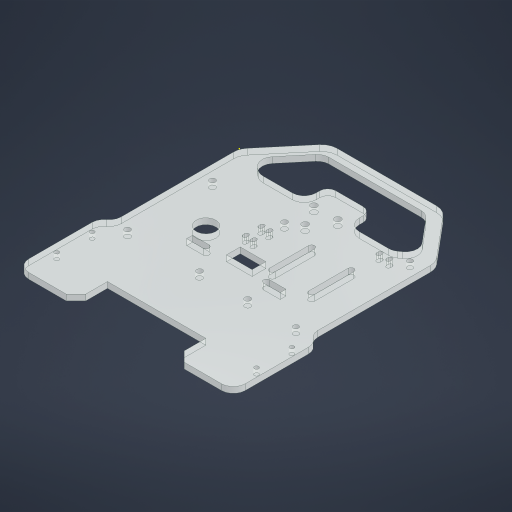
# Autodesk Inventor part: ROBOT CHASSIS PLATE
Saved by Autodesk Inventor 2023 (Build 270158000, 158)
## iProperties
Created: 2023-03-03
Part Number: ROBOT CHASSIS PLATE
Material: Generic
Document SubType Name: Modeling
Designer: Phoenix
Density: 1 g/cm^3
Appearance: Clear
Author: Phoenix
Autodesk Inventor part; units mm, degrees
note: some values were not read from the file. Chosen so that the rebuilt part matches the saved one: sketch regions of "Extrusion1"; arc direction of "Extrusion1".
ref_plane "YZ Plane" through (0, 0, 0) normal (1, 0, 0) x (0, 1, 0)
ref_plane "XZ Plane" through (0, 0, 0) normal (0, 1, 0) x (-1, 0, 0)
ref_plane "XY Plane" through (0, 0, 0) normal (0, 0, 1) x (1, 0, 0)
sketch "Sketch1" plane through (0, 0, 0) normal (0, 1, 0) x (-1, 0, 0)
  line L0 (0, 0) -> (-100, 0) construction
  line L1 (-100, 0) -> (-100, 100)
  line L2 (-100, 100) -> (0, 100)
  line L3 (0, 100) -> (0, 0)
  circle A0 centre (0.75, 92) radius 1.1
  circle A1 centre (0.75, 74) radius 1.1
  line L4 (-50, 100) -> (-50, 0) construction
  line L5 (-7.212, 20.82) -> (-7.212, 64) construction
  line L6 (-7.212, 64) -> (-43.788, 64) construction
  line L7 (-7.212, 20.82) -> (-43.788, 20.82) construction
  circle A2 centre (-7.212, 64) radius 1.5
  circle A3 centre (-43.788, 64) radius 1.5
  circle A4 centre (-7.212, 20.82) radius 1.5
  circle A5 centre (-43.788, 20.82) radius 1.5
  line L8 (-43.788, 6) -> (-92.788, 6) construction
  line L9 (-92.788, 6) -> (-92.788, 64) construction
  line L10 (-92.788, 64) -> (-43.788, 64) construction
  line L11 (-43.788, 64) -> (-43.788, 6) construction
  circle A6 centre (-43.788, 6) radius 1.375
  circle A7 centre (-92.788, 6) radius 1.375
  circle A8 centre (-92.788, 64) radius 1.375
  circle A9 centre (-43.788, 64) radius 1.375
  line L12 (-7.212, 42.41) -> (0, 42.41) construction
  line L13 (-92.788, 35) -> (-100, 35) construction
  line L14 (0, 0) -> (-100, 0) construction
  circle A10 centre (-100.75, 74) radius 1.1
  circle A11 centre (-100.75, 92) radius 1.1
  line L15 (-39, 6) -> (-61, 6)
  line L16 (-61, 6) -> (-61, -6)
  line L17 (-61, -6) -> (-39, -6)
  line L18 (-39, -6) -> (-39, 6)
  line L19 (-39, 6) -> (-61, -6) construction
  line L20 (-61, 6) -> (-39, -6) construction
  line L21 (-50, 0) -> (-50, -25) construction
  line L22 (-50, -25) -> (-20.9775, -25)
  line L23 (-20.9775, -25) -> (0, 0)
  line L24 (-7.8324, 0) -> (-23.7753, -19)
  line L25 (-23.7753, -19) -> (-50, -19)
  line L26 (-39, 6) -> (-16.1201, 6)
  line L27 (-16.1201, 6) -> (-7.8324, 0)
  line L28 (-50, -25) -> (-79.0225, -25)
  line L29 (-79.0225, -25) -> (-100, 0)
  line L30 (-92.1676, 0) -> (-76.2247, -19)
  line L31 (-76.2247, -19) -> (-50, -19)
  line L32 (-61, 6) -> (-83.8799, 6)
  line L33 (-83.8799, 6) -> (-92.1676, 0)
  line L34 (-30, 100) -> (-70, 100)
  line L35 (-50, -1) -> (-50, 12.462) construction
  circle A12 centre (-50, -1) radius 1.15 construction
  circle A13 centre (-50, 12.462) radius 1.15 construction
  circle A14 centre (-50, 9.5) radius 7 construction
  circle A15 centre (-50, 16.5) radius 1.65
  line L36 (0, 100) -> (5, 100)
  line L37 (5, 100) -> (5, 66)
  line L38 (5, 66) -> (0, 66)
  line L39 (0, 66) -> (0, 100)
  line L40 (-100, 100) -> (-105, 100)
  line L41 (-105, 100) -> (-105, 66)
  line L42 (-105, 66) -> (-100, 66)
  line L43 (5, 100) -> (-25, 100)
  line L44 (-25, 100) -> (-25, 108)
  line L45 (-25, 108) -> (5, 108)
  line L46 (5, 108) -> (5, 100)
  line L47 (-75, 100) -> (-75, 108)
  line L48 (-75, 108) -> (-105, 108)
  line L49 (-105, 108) -> (-105, 100)
  line L50 (-25, 100) -> (-75, 100)
  line L51 (-75, 100) -> (-75, 92)
  line L52 (-75, 92) -> (-25, 92)
  line L53 (-25, 92) -> (-25, 100)
  circle A16 centre (-56.0622, 6) radius 1.65
  circle A17 centre (-43.9378, 6) radius 1.65
  point P0 (-50, 80)
  point P1 (-50, 5.731)
  point P2 (-86.6667, 100)
  point P3 (-100, 92.8047)
  point P4 (-100, 91.1953)
  point P5 (-100, 74.8047)
  point P6 (-100, 73.1953)
  point P7 (0, 73.1953)
  point P8 (0, 74.8047)
  point P9 (0, 91.1953)
  point P10 (0, 92.8047)
  dimension "d27" = 3
  dimension "d47" = 14
  dimension "d0" = 100
  dimension "d1" = 100
  dimension "d2" = 8
  dimension "d4" = 2.2
  dimension "d5" = 18
  dimension "d6" = 43.18
  dimension "d7" = 36.576
  dimension "d8" = 3
  dimension "d9" = 49
  dimension "d10" = 58
  dimension "d15" = 2.75
  dimension "d33" = 22
  dimension "d34" = 25
  dimension "d36" = 130
  dimension "d37" = 6
  dimension "d38" = 6
  dimension "d39" = 12
  dimension "d44" = 2.3
  dimension "d45" = 13.462
  dimension "d46" = 5
  dimension "d48" = 15.5
  dimension "d49" = 3.3
  dimension "d55" = 5
  dimension "d56" = 34
  dimension "d57" = 4.25
  dimension "d59" = 30
  dimension "d60" = 8
  dimension "d61" = 8
  dimension "d64" = 360
  constraints: 108 end point, 17 centre point, 15 parallel, 13 symmetric about line, 11 coincident, 11 horizontal, 10 perpendicular, 10 point on line, 8 equal radius, 7 midpoint, 3 vertical, 1 vertical alignment, 11 other
  measures "d0" distance of L1.end L2.end
  measures "d1" distance of L0.end L1.end
  measures "d2" distance from line of L2 point (0.75, 92)
  measures "d4" diameter of A0
  measures "d5" distance of A0.centre A1.centre
  measures "d6" distance of L5.end L5.start
  measures "d7" distance of L5.end L6.end
  measures "d8" diameter of A2
  measures "d9" distance of L6.end L9.end
  measures "d10" distance of L8.end L9.end
  measures "d15" diameter of A8
  measures "d33" distance of L17.end L16.end
  measures "d34" distance of L4.end L21.end
  measures "d36" angle of L0 L23
  measures "d37" distance between parallel lines of L23 L24
  measures "d38" distance between parallel lines of L22 L25
  measures "d39" distance of L17.end L15.start
  measures "d44" diameter of A12
  measures "d45" distance of L35.end L35.start
  measures "d46" distance from line of L17 A12.centre
  measures "d48" distance from line of L17 point (-50, 9.5)
  measures "d49" diameter of A15
  measures "d55" distance of L37.end L38.end
  measures "d56" distance of L36.end L37.end
  measures "d57" distance from line of L37 A0.centre
  measures "d59" distance of L44.end L45.end
  measures "d60" distance of L43.end L44.end
  measures "d61" distance of L51.end L47.start
extrude "Extrusion1" add sketch "Sketch1" along normal blind 3 contours L1 A10 A11 L2 L51 L52 L53 L3 A0 A1 L23 L22 L28 L29 | L42 L41 L40 L1 A11 A10 | L49 L48 L47 L2 L40 | L3 A1 A0 L36 L37 L38 | L36 L2 L44 L45 L46 | L15 L18 L17 L16 A16 A17
fillet "Fillet1" radius 6 8 edges at (61, 1.5, 6) (39, 1.5, 6) (7.8324, 1.5, 0) (92.1676, 1.5, 0) (83.8799, 1.5, 6) (16.1201, 1.5, 6) (23.7753, 1.5, -19) (76.2247, 1.5, -19)
fillet "Fillet1" radius 8 4 edges at (20.9775, 1.5, -25) (0, 1.5, 0) (79.0225, 1.5, -25) (100, 1.5, 0)
fillet "Fillet1" radius 4 2 edges at (61, 1.5, -6) (39, 1.5, -6)
fillet "Fillet1" radius 6 6 edges at (105, 1.5, 66) (100, 1.5, 66) (-5, 1.5, 66) (0, 1.5, 66) (-5, 1.5, 108) (105, 1.5, 108)
sketch "Sketch2" plane through (0, 3, 0) normal (0, 1, 0) x (1, 0, 0)
  point P0 (0, 0)
sketch "Sketch3" plane through (0, 3, 0) normal (0, 1, 0) x (1, 0, 0)
  circle A0 centre (43.788, -64) radius 1.5 projected
  circle A1 centre (92.788, -6) radius 1.375 projected
  line L0 (43.788, -64) -> (92.788, -64) construction
  line L1 (92.788, -64) -> (92.788, -6) construction
  line L2 (92.788, -6) -> (43.788, -6) construction
  line L3 (43.788, -6) -> (43.788, -64) construction
  line L4 (61.788, -25) -> (61.788, -45) construction
  line L5 (60.288, -25) -> (60.288, -45)
  line L6 (63.288, -45) -> (63.288, -25)
  arc A2 (63.288, -25) -> (60.288, -25) centre (61.788, -25) ccw
  arc A3 (60.288, -45) -> (63.288, -45) centre (61.788, -45) ccw
  line L7 (43.788, -35) -> (92.788, -35) construction
  line L8 (81.788, -25) -> (81.788, -45) construction
  line L9 (80.288, -25) -> (80.288, -45)
  line L10 (83.288, -45) -> (83.288, -25)
  arc A4 (83.288, -25) -> (80.288, -25) centre (81.788, -25) ccw
  arc A5 (80.288, -45) -> (83.288, -45) centre (81.788, -45) ccw
  line L11 (63.788, -35) -> (112.788, -35) construction
  line L12 (81.788, -10) -> (81.788, -11) construction
  line L13 (80.788, -10) -> (80.788, -11)
  line L14 (82.788, -11) -> (82.788, -10)
  arc A6 (82.788, -10) -> (80.788, -10) centre (81.788, -10) ccw
  arc A7 (80.788, -11) -> (82.788, -11) centre (81.788, -11) ccw
  line L15 (85.788, -10) -> (85.788, -11)
  arc A8 (85.788, -11) -> (87.788, -11) centre (86.788, -11) ccw
  line L16 (86.788, -10) -> (86.788, -11) construction
  line L17 (87.788, -11) -> (87.788, -10)
  arc A9 (87.788, -10) -> (85.788, -10) centre (86.788, -10) ccw
  line L18 (43.788, -36) -> (43.788, -37) construction
  line L19 (42.788, -36) -> (42.788, -37)
  line L20 (44.788, -37) -> (44.788, -36)
  arc A10 (44.788, -36) -> (42.788, -36) centre (43.788, -36) ccw
  arc A11 (42.788, -37) -> (44.788, -37) centre (43.788, -37) ccw
  line L21 (57, 6) -> (43, 6) construction
  line L22 (50, 6) -> (50, -92) construction
  line L23 (25, -92) -> (75, -92) construction
  line L24 (39.788, -6) -> (39.788, -64) construction
  line L25 (40.788, -37) -> (40.788, -36)
  line L26 (39.788, -36) -> (39.788, -37) construction
  arc A12 (40.788, -36) -> (38.788, -36) centre (39.788, -36) ccw
  line L27 (38.788, -36) -> (38.788, -37)
  arc A13 (38.788, -37) -> (40.788, -37) centre (39.788, -37) ccw
  arc A14 (44.788, -28) -> (42.788, -28) centre (43.788, -28) ccw
  arc A15 (40.788, -28) -> (38.788, -28) centre (39.788, -28) ccw
  line L28 (44.788, -29) -> (44.788, -28)
  arc A16 (42.788, -29) -> (44.788, -29) centre (43.788, -29) ccw
  line L29 (43.788, -28) -> (43.788, -29) construction
  line L30 (42.788, -28) -> (42.788, -29)
  arc A17 (38.788, -29) -> (40.788, -29) centre (39.788, -29) ccw
  line L31 (39.788, -28) -> (39.788, -29) construction
  line L32 (38.788, -28) -> (38.788, -29)
  line L33 (40.788, -29) -> (40.788, -28)
  circle A18 centre (7.212, -20.82) radius 1.5 construction
  line L34 (7.212, -20.82) -> (43.788, -20.82) construction
  line L35 (43.788, -20.82) -> (43.788, -64) construction
  line L36 (43.788, -64) -> (7.212, -64) construction
  line L37 (7.212, -64) -> (7.212, -20.82) construction
  circle A19 centre (25.5, -42.41) radius 5
  circle A20 centre (68.288, -64) radius 1.5
  line L38 (73.75, -53) -> (26.25, -53)
  line L39 (26.25, -53) -> (26.25, -50)
  line L40 (26.25, -50) -> (73.75, -50)
  line L41 (73.75, -50) -> (73.75, -53)
  line L42 (73.75, -53) -> (26.25, -50) construction
  line L43 (26.25, -53) -> (73.75, -50) construction
  line L44 (45.3152, -53) -> (52.8728, -53)
  line L45 (51.6228, -50) -> (44.0652, -50)
  line L46 (35.4581, -50) -> (64.5419, -50)
  line L47 (64.5419, -50) -> (64.5419, -53)
  line L48 (64.5419, -53) -> (35.4581, -53)
  line L49 (35.4581, -53) -> (35.4581, -50)
  line L50 (35.4581, -50) -> (64.5419, -50)
  line L51 (64.5419, -50) -> (64.5419, -43)
  line L52 (64.5419, -43) -> (35.4581, -43)
  line L53 (35.4581, -43) -> (35.4581, -50)
  line L54 (35.4581, -50) -> (64.5419, -50)
  line L55 (64.5419, -50) -> (64.5419, -50)
  line L56 (64.5419, -50) -> (35.4581, -50)
  line L57 (35.4581, -50) -> (35.4581, -50)
  line L58 (43.5, -43) -> (56.5, -43)
  line L59 (56.5, -43) -> (56.5, -50)
  line L60 (56.5, -50) -> (43.5, -50)
  line L61 (43.5, -50) -> (43.5, -43)
  line L62 (43.5, -43) -> (56.5, -50) construction
  line L63 (56.5, -43) -> (43.5, -50) construction
  line L64 (35.4581, -51.5) -> (64.5419, -51.5) construction
  line L65 (26.25, -50) -> (33.15, -50)
  line L66 (33.15, -50) -> (33.15, -53)
  line L67 (33.15, -53) -> (26.25, -53)
  line L68 (26.25, -53) -> (26.25, -50)
  line L69 (66.85, -50) -> (66.85, -53)
  circle A21 centre (34.65, -51.5) radius 1.5
  circle A22 centre (65.35, -51.5) radius 1.5
  point P0 (0, 0)
  point P1 (61.788, -35)
  point P2 (81.788, -35)
  point P3 (81.788, -10.5)
  point P4 (86.788, -10.5)
  point P5 (43.788, -36.5)
  point P6 (39.788, -35)
  point P7 (39.788, -36.5)
  point P8 (43.788, -28.5)
  point P9 (39.788, -28.5)
  point P10 (50, -51.5)
  point P11 (50, -46.5)
  point P12 (50, -51.5)
  point P13 (43.5, -43)
  point P14 (43.5, -50)
  point P15 (56.5, -50)
  point P16 (56.5, -43)
  point P17 (65.35, -50)
  point P18 (65.35, -53)
  point P19 (34.65, -53)
  point P20 (34.65, -50)
  dimension "d66" = 3
  dimension "d67" = 18
  dimension "d68" = 20
  dimension "d71" = 20
  dimension "d76" = 1
  dimension "d77" = 2
  dimension "d78" = 4
  dimension "d81" = 5
  dimension "d86" = 1
  dimension "d87" = 2
  dimension "d90" = 4
  dimension "d97" = 8
  dimension "d102" = 27
  dimension "d108" = 10
  dimension "d109" = 3
  dimension "d110" = 47.5
  dimension "d111" = 3
  dimension "d113" = 11
  dimension "d114" = 0
  dimension "d115" = 13
  dimension "d116" = 6.9
  dimension "d117" = 7
  constraints: 152 end point, 32 point on circle, 20 centre point, 20 equal length, 18 tangent, 15 midpoint, 12 horizontal, 10 point on line, 8 perpendicular, 7 collinear, 4 vertical, 2 symmetric about line, 66 other
  measures "d66" diameter of A3
  measures "d67" distance from line of L3 point (61.788, -35)
  measures "d68" distance of L4.end L4.start
  measures "d71" distance of L5.start L9.start
  measures "d76" distance of L12.start L12.end
  measures "d77" diameter of A7
  measures "d78" distance from line of L2 L12.start
  measures "d81" distance of L13.end L15.end
  measures "d86" distance of L18.start L18.end
  measures "d87" diameter of A11
  measures "d90" distance of L2.end L24.start
  measures "d97" distance of L20.end L28.end
  measures "d102" distance of L0.start L18.end
  measures "d108" diameter of A19
  measures "d109" diameter of A20
  measures "d110" distance of L39.end L40.end
  measures "d111" distance of L38.end L39.end
  measures "d113" distance between parallel lines of L0 L38
  measures "d114" distance between parallel lines of L46 L56
  measures "d115" distance of L59.end L60.end
  measures "d116" distance of L66.end L67.end
  measures "d117" distance between parallel lines of L56 L52
extrude "Extrusion2" cut sketch "Sketch3" against normal blind 3 contours A2 L6 L52 L5 | L52 L6 A3 L5 | L59 L40 L61 L52 | L40 L69 A22 | A22 L47 | L47 A22 | L40 L41 L38 L69 | L69 L38 A22 | A21 L66 L40 | A21 L49 | A21 L49 | L66 L38 L39 L40 | A21 L38 L66 | A4 L10 A5 L9 | A6 L14 A7 L13 | A9 L17 A8 L15 | A10 L20 A11 L19 | A13 L27 A12 L25 | L28 A16 L30 A14 | L33 A17 L32 A15 | A19 | A20
chamfer "Chamfer2" distance 5 angle 45 2 edges at (25, 1.5, 108) (75, 1.5, 108)
body "Solid1"
